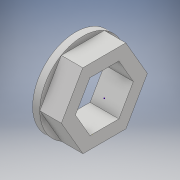
# Autodesk Inventor part: OuterLayerHub
Saved by Autodesk Inventor 2018 (Build 220112000, 112)
## iProperties
Created: 2019-06-04
Part Number: OuterLayerHub
Material: Generic
Document SubType Name: Modeling
Designer: Aditya Kendre
Density: 1 g/cm^3
Appearance: Default
Author: Aditya Kendre
Autodesk Inventor part; units mm, degrees
ref_plane "YZ Plane" through (0, 0, 0) normal (1, 0, 0) x (0, 1, 0)
ref_plane "XZ Plane" through (0, 0, 0) normal (0, 1, 0) x (-1, 0, 0)
ref_plane "XY Plane" through (0, 0, 0) normal (0, 0, 1) x (1, 0, 0)
sketch "Sketch1" plane through (0, 0, 0) normal (1, 0, 0) x (0, 1, 0)
  line L0 (0, 0) -> (3, 0) construction
  line L1 (3, 0) -> (3, -15.0663) construction
  line L2 (3, -15.0663) -> (0, -15.0663) construction
  line L3 (0, -15.0663) -> (0, 0) construction
  line L4 (0, 0) -> (-3, 0) construction
  line L5 (-3, 0) -> (-3, -15.0663) construction
  line L6 (-3, -15.0663) -> (0, -15.0663) construction
  line L7 (0, -15.0663) -> (0, 0) construction
  line L8 (3, -5.1752) -> (-2.9818, -5.1857)
  line L9 (-2.9818, -5.1857) -> (-5.9818, -0.0105)
  line L10 (-5.9818, -0.0105) -> (-3, 5.1752)
  line L11 (-3, 5.1752) -> (2.9818, 5.1857)
  line L12 (2.9818, 5.1857) -> (5.9818, 0.0105)
  line L13 (5.9818, 0.0105) -> (3, -5.1752)
  dimension "d0" = 3
  dimension "d1" = 3
  constraints: 28 end point, 4 parallel, 2 horizontal, 2 perpendicular, 1 coincident, 1 point on line, 13 other
  measures "d0" distance of L1.end L2.end
  measures "d1" distance of L6.end L5.end
extrude "Extrusion1" add sketch "Sketch1" along normal blind 3
sketch "Sketch2" plane through (0, 0, 0) normal (-1, 0, 0) x (0, 0, 1)
  point P0 (0, 0)
sketch "Sketch3" plane through (0, 0, 0) normal (-1, 0, 0) x (0, 0, 1)
  line L0 (-5.1752, 3) -> (0.0105, 5.9818) projected
  circle A0 centre (0, 0) radius 5.9818
  constraints: 1 coincident, 3 other
extrude "Extrusion2" add sketch "Sketch3" along normal blind 1
sketch "Sketch4" plane through (3, 0, 0) normal (1, 0, 0) x (0, 0, -1)
  line L0 (0, -4.0315) -> (-3.4914, -2.0157) construction
  line L1 (-3.4914, -2.0157) -> (-3.4914, 2.0157) construction
  line L2 (-3.4914, 2.0157) -> (0, 4.0315) construction
  line L3 (0, 4.0315) -> (3.4914, 2.0157) construction
  line L4 (3.4914, 2.0157) -> (3.4914, -2.0157) construction
  line L5 (3.4914, -2.0157) -> (0, -4.0315) construction
  point P0 (0, 0)
  point P1 (0, 0)
  constraints: 12 end point, 1 coincident, 13 other
sketch "Sketch5" plane through (3, 0, 0) normal (1, 0, 0) x (0, 0, -1)
  line L0 (0, -4.0314) -> (-3.4913, -2.0157)
  line L1 (-3.4913, -2.0157) -> (-3.4913, 2.0157)
  line L2 (-3.4913, 2.0157) -> (0, 4.0314)
  line L3 (0, 4.0314) -> (3.4913, 2.0157)
  line L4 (3.4913, 2.0157) -> (3.4913, -2.0157)
  line L5 (3.4913, -2.0157) -> (0, -4.0314)
  point P0 (0, 0)
  point P1 (0, 0)
  constraints: 12 end point, 1 coincident, 13 other
extrude "Extrusion3" cut sketch "Sketch5" against normal blind 10
body "Solid1"
